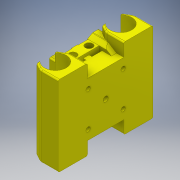
# Autodesk Inventor part: X Carriage
Saved by Autodesk Inventor 2016 (Build 200138000, 138)
## iProperties
Created: 2017-02-03
Part Number: X Carriage
Material: PC/ABS Plastic
Document SubType Name: Modeling
Designer: Scott
Density: 0.357273 g/cm^3
Appearance: Smooth - Yellow
Author: Scott
## iProperties of the stored document X Carriage_3DPrint.ipt
Created: 2017-03-27
Part Number: X Carriage_3DPrint
Material: Generic
Document SubType Name: Modeling
Designer: Scott
Density: 1 g/cm^3
Appearance: Default
Author: Scott
Autodesk Inventor part; units mm, degrees
ref_plane "YZ Plane" through (0, 0, 0) normal (1, 0, 0) x (0, 1, 0)
ref_plane "XZ Plane" through (0, 0, 0) normal (0, 1, 0) x (-1, 0, 0)
ref_plane "XY Plane" through (0, 0, 0) normal (0, 0, 1) x (1, 0, 0)
sketch "Sketch1" plane through (0, 0, 0) normal (0, 0, 1) x (1, 0, 0)
  arc A0 (-17.299765, 4.700235) -> (-17.299765, 15.299765) centre (-12, 10) ccw
  arc A1 (-17.299765, 49.700235) -> (-17.299765, 60.299765) centre (-12, 55) ccw
  arc A2 (-17.299765, 4.700235) -> (-17.299765, 15.299765) centre (-12, 10) ccw
  line L0 (0, 65) -> (0, 0)
  line L1 (-17.299765, 60.299765) -> (-17.299765, 62.299765)
  line L2 (0, 65) -> (-11.283076, 65)
  arc A3 (-11.283076, 65) -> (-13.783076, 64.330127) centre (-11.283076, 60) ccw
  line L3 (-17.299765, 62.299765) -> (-13.783076, 64.330127)
  line L4 (-17.299765, 4.700235) -> (-17.299765, 2.700235)
  line L5 (0, 0) -> (-11.283076, 0)
  arc A4 (-13.783076, 0.669873) -> (-11.283076, 0) centre (-11.283076, 5) ccw
  line L6 (-17.299765, 2.700235) -> (-13.783076, 0.669873)
  line L7 (-21.4, 49.700235) -> (-21.4, 15.299765)
  line L8 (-17.299765, 49.700235) -> (-21.4, 49.700235)
  line L9 (-21.4, 17.5) -> (-21.4, 22.5)
  line L10 (-17.299765, 15.299765) -> (-21.4, 15.299765)
  line L11 (-12, 10) -> (-17.299765, 4.700235) construction
  line L12 (-12, 10) -> (-17.299765, 15.299765) construction
  line L13 (-12, 10) -> (-27.848817, 10) construction
  line L14 (-12, 55) -> (-17.299765, 49.700235) construction
  line L15 (-12, 55) -> (-32.194667, 55) construction
  line L16 (-12, 55) -> (-17.299765, 60.299765) construction
  dimension "d0" = 65
  dimension "d1" = 12
  dimension "d2" = 12
  dimension "d3" = 45
  dimension "d4" = 7.495
  dimension "d5" = 7.495
  dimension "d6" = 21.4
  dimension "d7" = 5
  dimension "d8" = 5
  dimension "d10" = 45
  dimension "d11" = 45
  dimension "d12" = 45
  dimension "d13" = 2
  dimension "d14" = 2
  dimension "d15" = 30
  dimension "d16" = 30
  dimension "d17" = 10
  dimension "d18" = 10
  dimension "d19" = 42.5
  dimension "d20" = 47.5
  dimension "d21" = 27.84882
  dimension "d22" = 32.19467
  constraints: 34 end point, 10 point on circle, 6 tangent, 5 centre point, 3 parallel, 2 horizontal, 2 point on line, 1 coincident, 1 perpendicular, 1 vertical
  measures "d0" distance of L0.start L0.end
  measures "d1" distance from line of L14.start L0
  measures "d2" distance from line of L11.start L0
  measures "d3" distance of L11.start L14.start
  measures "d4" radius of A1
  measures "d5" radius of A0
  measures "d6" distance between parallel lines of L0 L7
  measures "d7" radius of A3
  measures "d8" radius of A4
  measures "d10" angle of L15 L16
  measures "d11" angle of L15 L14
  measures "d12" angle of L13 L12
  measures "d13" distance of L4.start L4.end
  measures "d14" distance of L1.start L1.end
  measures "d15" angle of L15 L3
  measures "d16" angle of L13 L6
  measures "d17" distance from line of L2 L14.start
  measures "d18" distance from line of L5 L11.start
  measures "d19" distance from line of L9.end L2
  measures "d20" distance from line of L9.start L2
  measures "d21" distance from line of L13.end L0
  measures "d22" distance from line of L15.end L0
extrude "Extrusion1" add sketch "Sketch1" along normal blind 55
ref_plane "Work Plane1" through (0, 0, 27.5) normal (0, 0, 1) x (1, 0, 0)
ref_plane "Work Plane2" through (-11.283076, 32.5, 0) normal (0, -1, 0) x (1, 0, 0)
sketch "Sketch2" plane through (0, 0, 55) normal (0, 0, 1) x (1, 0, 0)
  line L0 (-21.4, 15.299765) -> (-17.299765, 15.299765)
  line L1 (-17.299765, 49.700235) -> (-21.4, 49.700235)
  line L2 (-17.299765, 15.299765) -> (-17.299765, 17.299765)
  line L3 (-17.299765, 17.299765) -> (-13.783076, 19.330127)
  line L4 (-11.4, 19.998633) -> (-11.4, 45.001367)
  line L5 (-13.783076, 45.669873) -> (-17.299765, 47.700235)
  line L6 (-17.299765, 47.700235) -> (-17.299765, 49.700235)
  line L7 (0, 0) -> (0, 65)
  arc A0 (-17.299765, 4.700235) -> (-17.299765, 15.299765) centre (-12, 10) ccw
  arc A1 (-17.299765, 49.700235) -> (-17.299765, 60.299765) centre (-12, 55) ccw
  arc A2 (-11.4, 19.998633) -> (-13.783076, 19.330127) centre (-11.283076, 15) ccw
  arc A3 (-13.783076, 45.669873) -> (-11.4, 45.001367) centre (-11.283076, 50) ccw
  line L8 (-17.299765, 15.299765) -> (-21.4, 15.299765)
  line L9 (-21.4, 15.299765) -> (-21.4, 49.700235)
  line L10 (-21.4, 49.700235) -> (-17.299765, 49.700235)
  point P0 (-11.4, 20)
  point P1 (-11.4, 45)
  dimension "d27" = 2
  dimension "d28" = 2
  dimension "d31" = 11.4
  dimension "d34" = 5
  dimension "d103" = 120
  dimension "d104" = 120
  dimension "d105" = 11.28308
  dimension "d106" = 11.28308
  dimension "d107" = 4.70023
  dimension "d108" = 29.70023
  constraints: 16 end point, 4 point on circle, 3 point on line, 2 centre point, 2 collinear, 2 perpendicular, 2 tangent, 1 equal radius, 1 vertical
  measures "d27" distance of L0.end L2.end
  measures "d28" distance of L5.end L1.start
  measures "d31" distance between parallel lines of L7 L4
  measures "d34" radius of A2
  measures "d103" angle of L3 L2
  measures "d104" angle of L6 L5
  measures "d105" distance from line of A3.centre L7
  measures "d106" distance from line of A2.centre L7
  measures "d107" distance from line of point (-11.4, 45) L1
  measures "d108" distance from line of point (-11.4, 20) L1
extrude "Extrusion2" cut sketch "Sketch2" against normal blind 7
ref_plane "Work Plane3" through (0, 0, 29.5) normal (0, 0, 1) x (1, 0, 0)
sketch "Sketch3" plane through (0, 0, 29.5) normal (0, 0, 1) x (1, 0, 0)
  line L0 (4.28, 32.5) -> (-25.68, 32.5)
  line L1 (-11.4, 45.001367) -> (-11.4, 19.998633)
  line L2 (-11.4, 45.001367) -> (-11.4, 19.998633)
  line L3 (-13.4, 23.5) -> (-11.4, 23.5)
  line L4 (-11.4, 23.5) -> (-11.4, 30.5)
  line L5 (-11.4, 30.5) -> (-13.4, 30.5)
  line L6 (-13.4, 30.5) -> (-13.4, 23.5)
  line L7 (-13.4, 34.5) -> (-11.4, 34.5)
  line L8 (-11.4, 34.5) -> (-11.4, 41.5)
  line L9 (-11.4, 41.5) -> (-13.4, 41.5)
  line L10 (-13.4, 41.5) -> (-13.4, 34.5)
  point P0 (0, 0)
  point P1 (-11.4, 45)
  point P2 (-11.4, 20)
  dimension "d38" = 7
  dimension "d39" = 7
  dimension "d40" = 2
  dimension "d41" = 2
  dimension "d42" = 2
  constraints: 16 end point, 4 parallel, 3 point on line, 2 horizontal, 2 perpendicular
  measures "d38" distance of L5.end L3.start
  measures "d39" distance of L9.end L7.start
  measures "d40" distance between parallel lines of L0 L5
  measures "d41" distance between parallel lines of L0 L7
  measures "d42" distance of L3.start L3.end
extrude "Extrusion3" cut sketch "Sketch3" along normal through all
sketch "Sketch4" plane through (-21.4, 15.299765, 0) normal (-1, 0, 0) x (0, 0, 1)
  line L0 (29.5, 8.200235) -> (48, 8.200235)
  line L1 (29.5, 15.200235) -> (48, 15.200235)
  line L2 (29.5, 19.200235) -> (48, 19.200235)
  line L3 (29.5, 26.200235) -> (48, 26.200235)
  line L4 (29.5, 62.700235) -> (29.5, -28.299765)
  line L5 (29.5, 15.200235) -> (29.5, 8.200235)
  line L6 (29.5, 15.200235) -> (48, 15.200235)
  line L7 (29.5, 8.200235) -> (42, 8.200235)
  line L8 (42, 8.200235) -> (42, 15.200235)
  line L9 (42, 15.200235) -> (29.5, 15.200235)
  line L10 (29.5, 15.200235) -> (29.5, 8.200235)
  line L11 (29.5, 19.200235) -> (29.5, 26.200235)
  line L12 (29.5, 19.200235) -> (42, 19.200235)
  line L13 (42, 19.200235) -> (42, 26.200235)
  line L14 (42, 26.200235) -> (29.5, 26.200235)
  line L15 (29.5, 26.200235) -> (29.5, 19.200235)
  line L16 (48, 0) -> (48, 34.400469)
  point P0 (0, -15.299765)
  dimension "d45" = 6
  constraints: 16 end point, 4 parallel, 3 point on line, 2 horizontal, 2 perpendicular
  measures "d45" distance between parallel lines of L16 L8
extrude "Extrusion4" cut sketch "Sketch4" against normal up to surface (10 mm away) contours L4 L1 L8 L0 | L4 L3 L13 L2
sketch "Sketch5" plane through (0, 0, 48) normal (0, 0, 1) x (1, 0, 0)
  line L0 (-13.4, 23.5) -> (-13.4, 30.5)
  line L1 (-13.4, 34.5) -> (-13.4, 41.5)
  line L2 (-13.4, 27) -> (-25.86878, 27) construction
  line L3 (-13.4, 38) -> (-26.500916, 38) construction
  line L4 (-16.9, 24.519067) -> (-16.9, 40.494882) construction
  line L5 (-11.4, 45.001367) -> (-11.4, 19.998633) construction
  point P0 (0, 0)
  point P1 (-16.9, 27)
  point P2 (-16.9, 38)
  point P3 (-11.4, 45)
  point P4 (-11.4, 20)
  dimension "d48" = 5.5
  constraints: 6 end point, 4 point on line, 2 horizontal, 2 midpoint, 1 vertical
  measures "d48" distance between parallel lines of L5 L4
hole "Hole1" at (-16.9, 27, 48) at (-16.9, 38, 48) direction (0, 0, -1) diameter 4.7 depth 6 counterbore diameter 5 counterbore depth 0.5
sketch "Sketch7" plane through (-21.4, 15.299765, 0) normal (-1, 0, 0) x (0, 0, 1)
  line L0 (42, 15.200235) -> (42, 8.200235) construction
  line L1 (48, 0) -> (48, 34.400469) construction
  line L2 (42, 11.700235) -> (48, 17.200235) construction
  line L3 (45, 14.450235) -> (45, 39.825899) construction
  line L4 (45, 14.450235) -> (45, -5.049765) construction
  line L5 (66, 17.200235) -> (-11, 17.200235) construction
  point P0 (0, -15.299765)
  point P1 (45, 4.700235)
  point P2 (45, 29.700235)
  point P3 (45, 17.200235)
  dimension "d63" = 12.5
  dimension "d64" = 12.5
  constraints: 6 end point, 4 midpoint, 3 point on line, 2 vertical
  measures "d63" distance from line of L5 point (45, 4.7)
  measures "d64" distance from line of L5 point (45, 29.7)
hole "Hole3" at (-21.4, 20, 45) at (-21.4, 45, 45) direction (1, 0, 0) diameter 4.7 depth 5 counterbore diameter 5 counterbore depth 0.5
sketch "Sketch8" plane through (-21.4, 15.299765, 0) normal (-1, 0, 0) x (0, 0, 1)
  circle A0 centre (45, 4.700235) radius 2.5
  circle A1 centre (45, 29.700235) radius 2.5
  point P0 (0, -15.299765)
  constraints: 2 coincident
hole "Hole4" at (-21.4, 20, 45) at (-21.4, 45, 45) direction (1, 0, 0) diameter 3.5 depth 14
hole "Hole7" at (-21.4, 32.5, 45) direction (1, 0, 0) diameter 4.7 depth 6 counterbore diameter 5 counterbore depth 1.5
hole "Hole8" at (-21.4, 32.5, 45) direction (1, 0, 0) diameter 3.5 depth 7.6
sketch "Sketch9" plane through (-21.4, 30.5, 29.5) normal (0, -1, 0) x (1, 0, 0)
  line L0 (0, 12.5) -> (8, 12.5) construction
  line L1 (0, -29.5) -> (0, 18.5) construction
  line L2 (2, 18.5) -> (7, 18.5)
  line L3 (2, 18.5) -> (7, 18.5)
  line L4 (10, 18.5) -> (8, 18.5)
  line L5 (8, 18.5) -> (10, 18.5)
  line L6 (10, 18.5) -> (8, 18.5)
  line L7 (8, 18.5) -> (10, 18.5)
  line L8 (7.616924, 18.5) -> (10, 18.5)
  line L9 (4.100235, 18.5) -> (7.616924, 18.5)
  line L10 (0, 18.5) -> (4.100235, 18.5)
  line L11 (4.100235, 18.5) -> (0, 18.5)
  line L12 (7.616924, 18.5) -> (4.100235, 18.5)
  line L13 (10, 18.5) -> (7.616924, 18.5)
  line L14 (1.2, 12.5) -> (1.2, 18.5) construction
  line L15 (0.45, 12.5) -> (0.45, 12.759825)
  line L16 (0.210462, 13.5) -> (1.428329, 13.5) construction
  arc A0 (0.953803, 13.036181) -> (0.953803, 13.963819) centre (0.64, 13.5) ccw
  arc A1 (0.580435, 12.908543) -> (0.953803, 13.036181) centre (0.45, 13.9) ccw
  arc A2 (0.580435, 12.908543) -> (0.45, 12.759825) centre (0.6, 12.759825) ccw
  arc A3 (0.953803, 13.963819) -> (0.580435, 14.091457) centre (0.45, 13.1) ccw
  line L17 (0.45, 14.240175) -> (0.45, 14.5)
  arc A4 (0.45, 14.240175) -> (0.580435, 14.091457) centre (0.6, 14.240175) ccw
  line L18 (0, 12.5) -> (8, 12.5)
  line L19 (0.45, 12.5) -> (0, 12.5)
  line L20 (0, 12.5) -> (0, 14.5)
  line L21 (0, 13) -> (0, 18)
  line L22 (0, 14.5) -> (0.45, 14.5)
  point P0 (21.4, -29.5)
  point P1 (0.45, 12.9)
  point P2 (0.45, 14.1)
  dimension "d79" = 1.2
  dimension "d80" = 0.75
  dimension "d81" = 1.12
  dimension "d82" = 0.75
  dimension "d83" = 0.4
  dimension "d85" = 0.15
  dimension "d86" = 1
  dimension "d87" = 2
  dimension "d88" = 0.4
  dimension "d89" = 0
  dimension "d90" = 0.15
  dimension "d91" = 1
  dimension "d92" = 1
  constraints: 14 end point, 12 point on circle, 8 point on line, 5 centre point, 5 tangent, 2 perpendicular, 2 vertical, 1 collinear, 1 horizontal
  measures "d79" distance between parallel lines of L14 L1
  measures "d80" distance between parallel lines of L14 L15
  measures "d81" diameter of A0
  measures "d82" distance from line of L14 A1.centre
  measures "d83" distance from line of L16 A1.centre
  measures "d85" radius of A2
  measures "d86" distance between parallel lines of L0 L16
  measures "d87" diameter of A3
  measures "d88" distance from line of L16 A3.centre
  measures "d89" distance from line of L15 A3.centre
  measures "d90" radius of A4
  measures "d91" radius of A1
  measures "d92" distance between parallel lines of L16 L22
extrude "Extrusion5" cut sketch "Sketch9" along normal up to surface (7 mm away)
pattern_linear "Rectangular Pattern1" count 3 spacing 2 along (0, 0, 1) of "Extrusion5"
mirror "Mirror1" about plane through (-11.283076, 32.5, 0) normal (0, -1, 0) of "Extrusion5", "Rectangular Pattern1"
fillet "Fillet1" radius 5 2 edges at (-11.4, 27, 29.5) (-11.4, 38, 29.5)
sketch "Sketch10" plane through (-21.4, 15.299765, 0) normal (-1, 0, 0) x (0, 0, 1)
  line L0 (27.5, 62.700235) -> (27.5, -28.299765)
  line L1 (42, 19.200235) -> (42, 26.200235)
  line L2 (0, 34.400469) -> (48, 34.400469)
  line L3 (0, 0) -> (48, 0)
  line L4 (27.5, 0) -> (42, 0)
  line L5 (42, 0) -> (42, 34.400469)
  line L6 (42, 34.400469) -> (27.5, 34.400469)
  line L7 (27.5, 34.400469) -> (27.5, 0)
  point P0 (0, -15.299765)
  constraints: 8 end point, 3 point on line, 2 parallel, 1 collinear, 1 horizontal, 1 perpendicular
extrude "Extrusion6" cut sketch "Sketch10" against normal up to surface (4.100235 mm away)
mirror "Mirror2" about plane through (0, 0, 27.5) normal (0, 0, 1) of "Extrusion2", "Extrusion3", "Extrusion4", "Hole1", "Hole3", "Hole4", "Extrusion5", "Rectangular Pattern1", "Mirror1", "Fillet1", "Extrusion6", "Hole7", "Hole8"
sketch "Sketch11" plane through (0, 1, 0) normal (1, 0, 0) x (0, 0, -1)
  line L0 (11, 31.5) -> (-66, 31.5) projected
  line L1 (-27.5, -14) -> (-27.5, 77) projected
  line L2 (-39.5, 19.5) -> (-15.5, 19.5) construction
  line L3 (-15.5, 19.5) -> (-15.5, 43.5) construction
  line L4 (-15.5, 43.5) -> (-39.5, 43.5) construction
  line L5 (-39.5, 43.5) -> (-39.5, 19.5) construction
  point P0 (0, -1)
  point P1 (-39.5, 31.5)
  point P2 (-27.5, 19.5)
  dimension "d109" = 24
  dimension "d110" = 24
  dimension "d166" = 27.5
  dimension "d167" = 32.5
  constraints: 8 end point, 4 coincident, 2 midpoint, 2 parallel, 2 point on line, 1 horizontal, 1 perpendicular
  measures "d109" distance of L4.end L2.start
  measures "d110" distance of L3.end L4.end
  measures "d166" distance from line of point (0, -1) L1
  measures "d167" distance from line of point (0, -1) L0
hole "Hole6" at (0, 20.5, 39.5) at (0, 20.5, 15.5) at (0, 44.5, 15.5) at (0, 44.5, 39.5) direction (-1, 0, 0) diameter 3.05 depth 10
sketch "Sketch12" plane through (-21.4, 41.5, 48) normal (-1, 0, 0) x (0, 0, 1)
  line L0 (-6, 8.200235) -> (0, 8.200235)
  line L1 (-6, 8.200235) -> (-6, 0)
  line L2 (0, 0) -> (0, 8.200235)
  line L3 (-6, 8.200235) -> (0, 8.200235)
  line L4 (0, 8.200235) -> (2, 8.200235)
  line L5 (2, 8.200235) -> (2, 3.501367)
  line L6 (-6, 0) -> (0, 0)
  line L7 (-6, 0) -> (-8, 0)
  line L8 (-6, 0) -> (-18.5, 0)
  line L9 (-8, 8.200235) -> (-8, 0)
  line L10 (-35, 8.200235) -> (-6, 8.200235)
  line L11 (-8, 8.200235) -> (-6, 8.200235)
  line L12 (-6, -7) -> (-6, 0)
  line L13 (-6, 8.200235) -> (-6, 0)
  line L14 (0, 8.200235) -> (0, 6.200235)
  line L15 (0, 8.200235) -> (0, 0)
  circle A0 centre (-3, 3.5) radius 1.75
  line L16 (7, 3.501367) -> (0, 3.501367)
  line L17 (0, 0) -> (2, 3.501367)
  point P0 (-48, -41.5)
  dimension "d139" = 5
  dimension "d140" = 5
  constraints: 16 end point, 3 point on line, 2 collinear, 2 perpendicular, 1 horizontal, 1 vertical
  measures "d139" distance from line of L5 A0.centre
  measures "d140" distance from line of L9 A0.centre
extrude "Extrusion7" add sketch "Sketch12" against normal up to surface (10 mm away) contours L1 L7 L9 L10 | L4 L5 L16 L2 | L2 L16 L17
sketch "Sketch13" plane through (0, 0, 55) normal (0, 0, 1) x (1, 0, 0)
  arc A0 (-17.299765, 49.700235) -> (-17.299765, 60.299765) centre (-12, 55) ccw
  line L0 (-17.299765, 62.299765) -> (-17.299765, 60.299765)
  circle A1 centre (-12, 55) radius 7.495
  point P0 (0, 0)
  point P1 (-17.299765, 61.145065)
  constraints: 1 coincident, 3 other
extrude "Extrusion8" cut sketch "Sketch13" against normal blind 20
sketch "Sketch15" plane through (0, 65, 54) normal (1, 0, 0) x (0, 0, -1)
  line L0 (26.5, -78) -> (26.5, 13) projected
  line L1 (65, -32.5) -> (-12, -32.5) projected
  point P0 (54, -65)
  point P1 (26.5, -32.5)
  constraints: 2 midpoint
hole "Hole9" at (0, 32.5, 27.5) direction (-1, 0, 0) diameter 3.5 end through all
mirror "Mirror5" about plane through (-11.283076, 32.5, 0) normal (0, -1, 0) of "Extrusion7", "Extrusion8"
sketch "Sketch16" plane through (-13.4, 23.5, 42) normal (1, 0, 0) x (0, 0, -1)
  line L0 (-6, 0) -> (-8, -3.501367)
  line L1 (-13, -3.501367) -> (-8, -3.501367)
  line L2 (-13, -23.5) -> (-13, 41.5)
  line L3 (-13, 21.501367) -> (-8, 21.501367)
  line L4 (-8, 21.501367) -> (-6, 18)
  line L5 (7.5, 18) -> (-6, 18)
  line L6 (7.5, 0) -> (-6, 0)
  line L7 (-6, 0) -> (2, 0)
  line L8 (-4, 0) -> (-4, 18)
  point P0 (42, -23.5)
  dimension "d168" = 9
  constraints: 2 end point, 2 point on line, 1 vertical
  measures "d168" distance between parallel lines of L2 L8
extrude "Extrusion11" cut sketch "Sketch16" along normal through all
sketch "Sketch18" plane through (-20.95, 41.5, 42) normal (0, -1, 0) x (1, 0, 0)
  line L0 (9.55, 13) -> (9.55, 8) projected
  line L1 (9.55, 4) -> (20.95, 4) projected
  line L2 (9.55, 8) -> (20.95, 8) projected
  line L3 (20.95, 6) -> (20.95, 4) projected
  line L4 (20.95, 8) -> (20.95, 6) projected
  line L5 (9.55, 8) -> (15.95, 4)
  point P0 (20.95, -42)
  dimension "d176" = 5
  constraints: 2 end point, 1 point on line
  measures "d176" distance from line of L3 L5.end
extrude "Extrusion13" cut sketch "Sketch18" against normal up to surface (3.501367 mm away)
mirror "Mirror6" about plane through (-11.283076, 32.5, 0) normal (0, -1, 0) of "Extrusion13"
mirror "Mirror7" about plane through (0, 0, 27.5) normal (0, 0, 1) of "Extrusion11", "Extrusion13", "Mirror6", "Extrusion7", "Extrusion8", "Mirror5"
fillet "Fillet8" radius 1 24 edges at (-12.5772, 0.1704, 55) (-5.6415, 0, 55) (-15.5414, 1.6851, 55) (-5.7, 45.0014, 55) (-12.6336, 45.1858, 55) (-15.5414, 46.6851, 55) (-12.6336, 19.8142, 55) (-15.5414, 18.3149, 55) (-5.7, 19.9986, 55) (-12.5772, 64.8296, 55) (-15.5414, 63.3149, 55) (-5.6415, 65, 55) (-12.5772, 64.8296, 0) (-5.6415, 65, 0) (-15.5414, 63.3149, 0) (-12.6336, 45.1858, 0) (-15.5414, 46.6851, 0) (-12.6336, 19.8142, 0) (-15.5414, 18.3149, 0) (-12.5772, 0.1704, 0) (-5.6415, 0, 0) (-15.5414, 1.6851, 0) (-5.7, 45.0014, 0) (-5.7, 19.9986, 0)
fillet "Fillet9" radius 1 16 edges at (-19.3499, 15.2998, 50) (-19.3499, 15.2998, 40) (-19.3499, 23.5, 40) (-16.4, 19.9986, 50) (-16.4, 45.0014, 50) (-19.3499, 49.7002, 50) (-19.3499, 49.7002, 40) (-19.3499, 41.5, 40) (-19.3499, 15.2998, 15) (-19.3499, 15.2998, 5) (-19.3499, 23.5, 15) (-16.4, 19.9986, 5) (-16.4, 45.0014, 5) (-19.3499, 49.7002, 5) (-19.3499, 49.7002, 15) (-19.3499, 41.5, 15)
equation "\"d64\" = d63"
body "Solid1"
